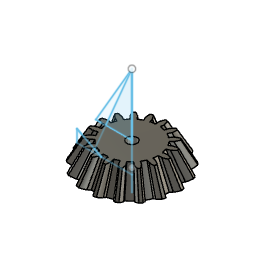
Small Gear (Autodesk Fusion 360 design; units mm, degrees)
Autodesk Fusion 360 part; units mm, degrees
sketch "sketch 1152" plane through (0, 32, 100) normal (0, 1, 0) x (1, 0, 0)
  line L0 (-9.1584, 21.6708) -> (-7.5, 22.5)
  line L1 (-9.1584, 21.6708) -> (-7.5, 22.5)
  line L2 (-9.1584, 21.6708) -> (0, 0)
  line L3 (0, 21) -> (0, 0)
  line L4 (0, 21.6708) -> (0, 21)
  line L5 (0, 22.5) -> (0, 21.6708)
  line L6 (-7.5, 22.5) -> (0, 22.5)
revolve "Revolve1" add sketch "sketch 1152" angle 360 about axis through (0, 32, 73.75) along (0, 0, 1) makes body 1
ref_plane "WorkPlane1" through (0, 40.3292, 77.9146) normal (0, 0.447214, -0.894427) x (-1, 0, 0)
sketch "Sketch1" plane through (0, 40.3292, 77.9146) normal (0, 0.447214, -0.894427) x (-1, 0, 0)
  line L0 (0, 0) -> (0, -11)
  line L1 (0, -11) -> (-0.909, 2)
  line L2 (0, -11) -> (0.909, 2)
  line L3 (-0.375, 3.5) -> (0.375, 3.5)
  arc A0 (-0.375, 3.5) -> (-0.909, 2) centre (3.5304, 1.2645) ccw
  arc A1 (0.909, 2) -> (0.375, 3.5) centre (-3.5304, 1.2645) ccw
  line L4 (0.8042, 0.5) -> (-0.8042, 0.5)
  dimension "d1011" = 11
  dimension "d1012" = 0.375
  dimension "d1013" = 0.75
  dimension "d1014" = 3.5
  dimension "d1015" = 13
  dimension "d1017" = 4
  dimension "d1018" = 4
  dimension "d1019" = 4.5
  dimension "d1020" = 0.5
  constraint coincident L0.start origin
  constraint vertical L0
  constraint horizontal L3
  constraint equal L1 L2
  constraint equal A0 A1
  constraint coincident L2 L4.start
  constraint coincident L1 L4.end
  constraint horizontal L4
  measures "d1011" distance of L0.start L0.end
  measures "d1012" horizontal distance of L0.start L3.end
  measures "d1013" distance of L3.start L3.end
  measures "d1014" distance of L0.start L3
  measures "d1015" vertical distance of L0.end L2.end
  measures "d1017" angle of L0 L2
  measures "d1018" angle of L0 L1
  measures "d1019" radius of A1
  measures "d1020" distance of L0.start L4
loft "Loft1" add profiles "Sketch1" section 1 contours L1 L2 L3 A0 A1 L4 section 2 point at (0, 32, 100) separate body makes body 2
pattern_circular "C-Pattern1" count 17 over 360 about axis through (0, 32, 79) along (0, 0, 1) of bodies 2 makes body 3 at (-2.1136, 37.4558, 85.4255) makes body 4 at (-3.9417, 36.3239, 85.4255) makes body 5 at (-5.2375, 34.608, 85.4255) makes body 6 at (-5.826, 32.5399, 85.4255) makes body 7 at (-5.6276, 30.3988, 85.4255) makes body 8 at (-4.6691, 28.474, 85.4255) makes body 9 at (-3.0801, 27.0254, 85.4255) makes body 10 at (-1.0751, 26.2487, 85.4255) makes body 11 at (1.0751, 26.2487, 85.4255) makes body 12 at (3.0801, 27.0254, 85.4255) makes body 13 at (4.6691, 28.474, 85.4255) makes body 14 at (5.6276, 30.3988, 85.4255) makes body 15 at (5.826, 32.5399, 85.4255) makes body 16 at (5.2375, 34.608, 85.4255) makes body 17 at (3.9417, 36.3239, 85.4255) makes body 18 at (2.1136, 37.4558, 85.4255)
sketch "sketch 1179" plane through (0, 32, 100) normal (0, 1, 0) x (1, 0, 0)
  line L0 (0, 26.25) -> (0, 22.5)
  line L1 (0, 21) -> (0, 0)
  line L2 (-6.4334, 15.223) -> (-7.6115, 15.223)
  line L3 (-7.6115, 15.223) -> (-8.8673, 15.223)
  line L4 (-8.8673, 15.223) -> (0, 0)
  line L5 (0, 15.223) -> (0, 0)
  line L6 (-6.4334, 15.223) -> (0, 15.223)
  line L7 (-10.5, 21) -> (-9.1584, 21.6708)
  line L8 (-9.1584, 21.6708) -> (-7.5, 22.5)
  line L9 (-9.1584, 21.6708) -> (-7.5, 22.5)
  line L10 (-13.5, 22.5) -> (-7.5, 22.5)
  line L11 (-13.5, 19.5) -> (-13.5, 22.5)
  line L12 (-11.8416, 20.3292) -> (-13.5, 19.5)
  line L13 (-10.5, 21) -> (-11.8416, 20.3292)
  line L14 (-10.5, 21) -> (-11.8416, 20.3292)
  line L15 (0, 26.25) -> (0, 22.5)
revolve "Revolve3" cut sketch "sketch 1179" angle 360 about axis through (0, 32, 73.75) along (0, 0, 1) bodies 1 2 6 7 8 4 5 3 12 13 17 15 10 11 9 16 14 18
combine "Combine1" operation add target body 1 tool bodies 2 6 7 8 4 5 3 12 13 17 15 10 11 9 16 14 18
hole "Hole1" at (0, 32, 77.5) direction (0, 0, 1) diameter 2.5 depth 7.5 tip angle 118 bodies 1
equation "d1012 = d1013 / 2"
equation "d1021 = 34 / 2"
named bodies: "Small Gear"
